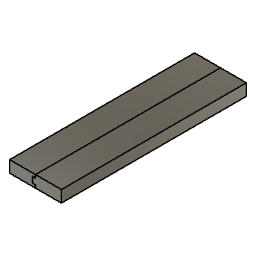
Tongue and Groove Joint (Autodesk Fusion 360 design; units mm, degrees)
Autodesk Fusion 360 part; units mm, degrees
sketch "Base" plane through (0, 0, 0) normal (1, 0, 0) x (0, 1, 0)
  line L0 (-40, 50) -> (260, 50)
  line L1 (260, 50) -> (260, 31)
  line L2 (260, 31) -> (-40, 31)
  line L3 (-40, 31) -> (-40, 50)
  dimension "d4" = 300
  dimension "d5" = 19
  constraint horizontal L0
  constraint vertical L1
  constraint horizontal L2
  constraint vertical L3
  measures "d4" distance of L0.start L0.end
  measures "d5" distance of L0.start L2.end
extrude "Extrude1" add sketch "Base" against normal blind 42 makes body 1
copy_body "Body->Comp1" bodies 1 removing the originals makes body 2 in component "First Piece"
sketch "Cut" plane through (0, 0, 0) normal (1, 0, 0) x (0, 1, 0)
  line L0 (-40, 31) -> (260, 31)
  line L1 (260, 31) -> (260, 50)
  line L2 (260, 50) -> (-40, 50)
  line L3 (-40, 50) -> (-40, 31)
  line L4 (-40, 45.25) -> (260, 45.25)
  line L5 (260, 45.25) -> (260, 35.75)
  line L6 (260, 35.75) -> (-40, 35.75)
  line L7 (-40, 35.75) -> (-40, 45.25)
  dimension "d8" = 300
  dimension "d9" = 9.5
  constraint horizontal L4
  constraint vertical L5
  constraint horizontal L6
  constraint vertical L7
  constraint coincident L3 L4.start
  constraint midpoint L1 L5
  measures "d8" distance of L4.start L4.end
  measures "d9" distance of L4.start L6.end
extrude "Extrude1'" cut sketch "Cut" against normal blind 5 contours L1 L3 L4 L5 L6 L7 bodies 2 in component "First Piece"
extrude "Extrude1''" add sketch "Cut" against normal blind 5 separate body contours L1 L3 L4 L5 L6 L7 makes body 3 in component "Second Piece"
extrude "Extrude2" add sketch "Cut" along normal blind 42 bodies 3 in component "Second Piece"
component "First Piece" placed x (1, 0, 0) y (0, 1, 0) z (0, 0, 1) at (0, 0, 0)
component "Second Piece" placed x (1, 0, 0) y (0, 1, 0) z (0, 0, 1) at (0, 0, 0)
equation "length = 300 mm"
equation "width = 42 mm"
equation "thickness = 19 mm"
equation "d4 = length"
equation "d5 = thickness"
equation "d6 = -width"
equation "d8 = length"
equation "d9 = thickness / 2"
equation "d14 = width"
named bodies: "First Piece", "Second Piece"
